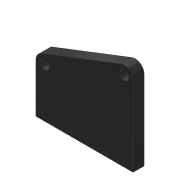
# Autodesk Inventor part: COXA_ROLL_COUPLER_BACK
Saved by Autodesk Inventor 2019.4 (Build 234330000, 330)
## iProperties
Created: 2019-10-21
Part Number: COXA_ROLL_COUPLER_BACK
Material: 一般
Document SubType Name: Modeling
Designer: y6tada
Density: 1 g/cm^3
Appearance: 濃い灰色
Author: y6tada
Autodesk Inventor part; units mm, degrees
ref_plane "YZ Plane" through (0, 0, 0) normal (1, 0, 0) x (0, 1, 0)
ref_plane "XZ Plane" through (0, 0, 0) normal (0, 1, 0) x (-1, 0, 0)
ref_plane "XY Plane" through (0, 0, 0) normal (0, 0, 1) x (1, 0, 0)
sketch "スケッチ1" plane through (0, 0, 0) normal (0, 0, 1) x (1, 0, 0)
  line L0 (0, 0) -> (36, 13.862) construction
  line L1 (34.5627, 17.5948) -> (-1.4373, 3.7328)
  line L2 (-4, 0) -> (-4, -22.2053)
  line L3 (-4, -22.2053) -> (40, -22.2053)
  line L4 (40, -22.2053) -> (40, 13.862)
  arc A0 (-1.4373, 3.7328) -> (-4, 0) centre (0, 0) ccw
  arc A1 (40, 13.862) -> (34.5627, 17.5948) centre (36, 13.862) ccw
  dimension "d0" = 36
  dimension "d1" = 13.862
  dimension "d2" = 4
  constraints: 10 end point, 4 coincident, 4 point on circle, 4 tangent, 2 centre point, 2 perpendicular, 1 equal radius, 1 horizontal
  measures "d0" horizontal distance of L0.end point (0, 0)
  measures "d1" vertical distance of point (0, 0) L0.end
  measures "d2" radius of A0
extrude "押し出し1" add sketch "スケッチ1" along normal blind 5
hole "穴1" at (0, 0, 0) at (36, 13.862, 0) direction (0, 0, 1) diameter 4 end through all
